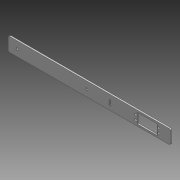
# Autodesk Inventor part: extension
Saved by Autodesk Inventor 2016 (Build 200138000, 138)
## iProperties
Created: 2019-01-31
Part Number: extension
Material: Generic
Document SubType Name: Modeling
Designer: TYP
Density: 1 g/cm^3
Appearance: Default
Author: TYP
Autodesk Inventor part; units mm, degrees
ref_plane "YZ Plane" through (0, 0, 0) normal (1, 0, 0) x (0, 1, 0)
ref_plane "XZ Plane" through (0, 0, 0) normal (0, 1, 0) x (-1, 0, 0)
ref_plane "XY Plane" through (0, 0, 0) normal (0, 0, 1) x (1, 0, 0)
sketch "Sketch1" plane through (0, 0, 0) normal (0, 1, 0) x (-1, 0, 0)
  line L0 (-3, -15) -> (-347, -15)
  line L1 (-350, -12) -> (-350, 12)
  line L2 (-347, 15) -> (-3, 15)
  line L3 (0, 12) -> (0, -12)
  line L4 (0, 0) -> (-350, 0) construction
  circle A0 centre (-20, 0) radius 2.25
  circle A1 centre (-170, 0) radius 2.25
  line L5 (-278.75, -11) -> (-321.25, -11)
  line L6 (-321.25, -11) -> (-321.25, 11)
  line L7 (-321.25, 11) -> (-278.75, 11)
  line L8 (-278.75, 11) -> (-278.75, -11)
  line L9 (-278.75, 0) -> (-321.25, 0) construction
  line L10 (-278.75, -2.5) -> (-278.75, 2.5)
  line L11 (-275.25, 5) -> (-324.75, 5) construction
  line L12 (-324.75, 5) -> (-324.75, -5) construction
  line L13 (-324.75, -5) -> (-275.25, -5) construction
  line L14 (-275.25, -5) -> (-275.25, 5) construction
  line L15 (-324.75, 5) -> (-275.25, -5) construction
  line L16 (-324.75, -5) -> (-275.25, 5) construction
  circle A2 centre (-275.25, -5) radius 2.25
  circle A3 centre (-275.25, 5) radius 2.25
  circle A4 centre (-324.75, -5) radius 2.25
  circle A5 centre (-324.75, 5) radius 2.25
  arc A6 (-3, -15) -> (0, -12) centre (-3, -12) ccw
  arc A7 (0, 12) -> (-3, 15) centre (-3, 12) ccw
  arc A8 (-347, 15) -> (-350, 12) centre (-347, 12) ccw
  arc A9 (-350, -12) -> (-347, -15) centre (-347, -12) ccw
  point P0 (0, -15)
  point P1 (-350, 15)
  point P2 (-350, -15)
  point P3 (0, 15)
  point P4 (-305.045, 0)
  point P5 (-300, 0)
  dimension "d0" = 350
  dimension "d1" = 30
  dimension "d3" = 20
  dimension "d5" = 150
  dimension "d6" = 22
  dimension "d7" = 42.5
  dimension "d8" = 300
  dimension "d10" = 5
  dimension "d13" = 10
  dimension "d14" = 49.5
  dimension "d15" = 2.25
  dimension "d16" = 2.25
  dimension "d17" = 2.25
  dimension "d18" = 2.25
  dimension "d21" = 3
  dimension "d22" = 4.5
  dimension "d23" = 4.5
  constraints: 34 end point, 12 point on line, 10 centre point, 8 point on circle, 8 tangent, 7 midpoint, 6 parallel, 5 coincident, 3 equal radius, 3 horizontal, 3 perpendicular
  measures "d0" distance of point (-350, 15) point (0, 15)
  measures "d1" distance of point (0, 15) point (0, -15)
  measures "d3" distance from line of L3 A0.centre
  measures "d5" distance of A0.centre A1.centre
  measures "d6" distance of L7.end L5.start
  measures "d7" distance of L6.end L7.end
  measures "d8" distance from line of point (-300, 0) L3
  measures "d10" distance of L10.start L10.end
  measures "d13" distance of L11.end L12.end
  measures "d14" distance of L11.start L11.end
  measures "d15" radius of A2
  measures "d16" radius of A3
  measures "d17" radius of A4
  measures "d18" radius of A5
  measures "d21" radius of A6
  measures "d22" diameter of A1
  measures "d23" diameter of A0
extrude "Extrusion1" add sketch "Sketch1" along normal blind 3
sketch "Sketch2" plane through (0, 0, 0) normal (0, -1, 0) x (1, 0, 0)
  line L0 (221.5, 5) -> (218.5, 5)
  line L1 (218.5, 5) -> (218.5, -5)
  line L2 (218.5, -5) -> (221.5, -5)
  line L3 (221.5, -5) -> (221.5, 5)
  line L4 (221.5, 5) -> (218.5, -5) construction
  line L5 (218.5, 5) -> (221.5, -5) construction
  line L6 (0, -12) -> (0, 12) projected
  point P0 (0, 0)
  point P1 (220, 0)
  point P2 (220, 0)
  point P3 (0, 0)
  dimension "d24" = 3
  dimension "d25" = 10
  dimension "d26" = 220
  constraints: 12 end point, 4 midpoint, 2 parallel, 1 horizontal, 1 horizontal alignment, 1 perpendicular
  measures "d24" distance of L2.end L1.end
  measures "d25" distance of L1.end L0.end
  measures "d26" distance from line of L6 point (220, 0)
extrude "Extrusion2" cut sketch "Sketch2" against normal blind 10
body "Solid1"
